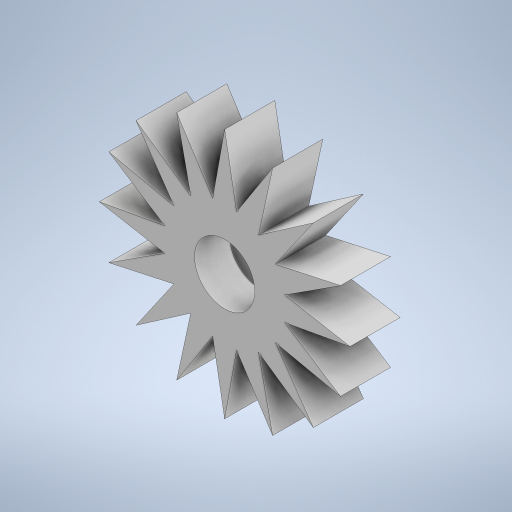
# Autodesk Inventor part: GEAR_SERV
Saved by Autodesk Inventor 2024.3 (Build 283343000, 343)
## iProperties
Created: 2024-07-29
Part Number: GEAR_SERV
Material: Ogólny
Document SubType Name: Modeling
Designer: User
Density: 1 g/cm^3
Appearance: Domyślna
Author: User
Autodesk Inventor part; units mm, degrees
ref_plane "YZ Plane" through (0, 0, 0) normal (1, 0, 0) x (0, 1, 0)
ref_plane "XZ Plane" through (0, 0, 0) normal (0, 1, 0) x (-1, 0, 0)
ref_plane "XY Plane" through (0, 0, 0) normal (0, 0, 1) x (1, 0, 0)
sketch "Szkic1" plane through (0, 0, 0) normal (0, 0, 1) x (1, 0, 0)
  circle A0 centre (0, 0) radius 2.25
  circle A1 centre (0, 0) radius 3
  dimension "d0" = 4.5
  dimension "d1" = 6
  constraints: 2 centre point, 2 coincident
  measures "d0" diameter of A0
  measures "d1" diameter of A1
extrude "Wyciągnięcie proste1" add sketch "Szkic1" against normal blind 1
sketch "Szkic4" plane through (0, 0, 0) normal (0, 0, 1) x (1, 0, 0)
  circle A0 centre (0, 0) radius 2.25 projected
  circle A1 centre (0, 0) radius 3 projected
  circle A2 centre (0, 0) radius 3
  circle A3 centre (0, 0) radius 2.25
  circle A4 centre (0, 0) radius 3.65
  line L0 (0, 0) -> (0, 8.5)
  circle A5 centre (0, 0) radius 2.4
  line L1 (0, 8.5) -> (0, 9.5)
  line L2 (0, 8.5) -> (5.1877, 8.5) construction
  line L3 (0, 9.5) -> (0, 10)
  line L4 (0, 10) -> (1.1899, 3.4506)
  line L5 (0, 10) -> (-1.1899, 3.4506)
  line L6 (-3.8268, 9.2388) -> (-0.2212, 3.6433)
  line L7 (-3.8268, 9.2388) -> (-2.4198, 2.7326)
  line L8 (-7.0711, 7.0711) -> (-1.5985, 3.2813)
  line L9 (-7.0711, 7.0711) -> (-3.2813, 1.5985)
  line L10 (-9.2388, 3.8268) -> (-2.7326, 2.4198)
  line L11 (-9.2388, 3.8268) -> (-3.6433, 0.2212)
  line L12 (-10, 0) -> (-3.4506, 1.1899)
  line L13 (-10, 0) -> (-3.4506, -1.1899)
  line L14 (-9.2388, -3.8268) -> (-3.6433, -0.2212)
  line L15 (-9.2388, -3.8268) -> (-2.7326, -2.4198)
  line L16 (-7.0711, -7.0711) -> (-3.2813, -1.5985)
  line L17 (-7.0711, -7.0711) -> (-1.5985, -3.2813)
  line L18 (-3.8268, -9.2388) -> (-2.4198, -2.7326)
  line L19 (-3.8268, -9.2388) -> (-0.2212, -3.6433)
  line L20 (0, -10) -> (-1.1899, -3.4506)
  line L21 (0, -10) -> (1.1899, -3.4506)
  line L22 (3.8268, -9.2388) -> (0.2212, -3.6433)
  line L23 (3.8268, -9.2388) -> (2.4198, -2.7326)
  line L24 (7.0711, -7.0711) -> (1.5985, -3.2813)
  line L25 (7.0711, -7.0711) -> (3.2813, -1.5985)
  line L26 (9.2388, -3.8268) -> (2.7326, -2.4198)
  line L27 (9.2388, -3.8268) -> (3.6433, -0.2212)
  line L28 (10, 0) -> (3.4506, -1.1899)
  line L29 (10, 0) -> (3.4506, 1.1899)
  line L30 (9.2388, 3.8268) -> (3.6433, 0.2212)
  line L31 (9.2388, 3.8268) -> (2.7326, 2.4198)
  line L32 (7.0711, 7.0711) -> (3.2813, 1.5985)
  line L33 (7.0711, 7.0711) -> (1.5985, 3.2813)
  line L34 (3.8268, 9.2388) -> (2.4198, 2.7326)
  line L35 (3.8268, 9.2388) -> (0.2212, 3.6433)
  point P0 (-0.9495, 4.7736)
  point P1 (-2.704, 4.0469)
  point P2 (-4.0469, 2.704)
  point P3 (-4.7736, 0.9495)
  point P4 (-4.7736, -0.9495)
  point P5 (-4.0469, -2.704)
  point P6 (-2.704, -4.0469)
  point P7 (-0.9495, -4.7736)
  point P8 (0.9495, -4.7736)
  point P9 (2.704, -4.0469)
  point P10 (4.0469, -2.704)
  point P11 (4.7736, -0.9495)
  point P12 (4.7736, 0.9495)
  point P13 (4.0469, 2.704)
  point P14 (2.704, 4.0469)
  point P15 (0.9495, 4.7736)
  dimension "d29" = 7.3
  dimension "d44" = 8.5
  dimension "d50" = 4.8
  dimension "d51" = 1
  dimension "d76" = 0.5
  dimension "d79" = 360
  constraints: 72 end point, 4 coincident, 3 centre point, 3 vertical, 2 concentric, 1 horizontal, 1 symmetric about line, 84 other
  measures "d44" distance of L0.start L0.end
  measures "d50" diameter of A5
  measures "d51" distance of L0.end L1.end
  measures "d76" distance of L1.end L3.end
extrude "Wyciągnięcie proste4" add sketch "Szkic4" along normal blind 4 contours A5 | A1 | A4 | A4 L6 L5 L3 L1 L0 | L0 L1 L3 L4 L35 A4 | L35 L4 A4 | A4 L5 L6 | L4 L35 L34 L33 A4 | A4 L8 L7 L6 L5 | L33 L34 A4 | A4 L7 L8 | L34 L33 L32 L31 A4 | A4 L10 L9 L8 L7 | L31 L32 A4 | A4 L9 L10 | L32 L31 L30 L29 A4 | A4 L12 L11 L10 L9 | L29 L30 A4 | A4 L11 L12 | L30 L29 L28 L27 A4 | A4 L14 L13 L12 L11 | A4 L13 L14 | L27 L28 A4 | L27 L26 L25 A4 L28 | A4 L16 L15 L14 L13 | A4 L15 L16 | L25 L26 A4 | L25 L24 L23 A4 L26 | A4 L18 L17 L16 L15 | A4 L17 L18 | L23 L24 A4 | L23 L22 L21 A4 L24 | A4 L20 L19 L18 L17 | A4 L19 L20 | L21 L22 A4 | L21 L20 L19 A4 L22
sketch "Szkic5" plane through (0, 0, 4) normal (0, 0, 1) x (1, 0, 0)
  circle A0 centre (0, 0) radius 2.35
  dimension "d41" = 4.7
  constraints: 1 centre point, 1 coincident
  measures "d41" diameter of A0
extrude "Wyciągnięcie proste5" cut sketch "Szkic5" against normal through all
sketch "Szkic6" plane through (0, 0, 4) normal (0, 0, 1) x (1, 0, 0)
  circle A0 centre (0, 0) radius 2.4
  dimension "d57" = 4.8
  constraints: 1 centre point, 1 coincident
  measures "d57" diameter of A0
extrude "Wyciągnięcie proste6" cut sketch "Szkic6" against normal through all
ref_plane "Płaszczyzna konstrukcyjna1" through (0, 0, 0) normal (0, 0, -1) x (-1, 0, 0)
sketch "Szkic7" plane through (0, 0, 0) normal (0, 0, -1) x (-1, 0, 0)
  circle A0 centre (0, 0) radius 2.4
  circle A1 centre (0, 0) radius 1.5
  dimension "d61" = 3
  constraints: 2 centre point, 2 coincident
  measures "d61" diameter of A1
extrude "Wyciągnięcie proste7" add sketch "Szkic7" against normal blind 1.2
